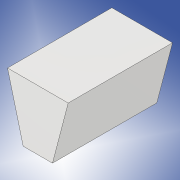
# Autodesk Inventor part: TA004
Saved by Autodesk Inventor 2017 (Build 210142000, 142)
## iProperties
Created: 2017-06-21
Part Number: TA004
Material: ABS Plastic
Document SubType Name: Modeling
Designer: zallen
Density: 1.06 g/cm^3
Appearance: CR White
Author: zallen
Autodesk Inventor part; units mm, degrees
ref_plane "YZ Plane" through (0, 0, 0) normal (1, 0, 0) x (0, 1, 0)
ref_plane "XZ Plane" through (0, 0, 0) normal (0, 1, 0) x (-1, 0, 0)
ref_plane "XY Plane" through (0, 0, 0) normal (0, 0, 1) x (1, 0, 0)
sketch "Sketch1" plane through (0, 0, 0) normal (0, 0, 1) x (1, 0, 0)
  line L0 (0, 0) -> (77.1779, 0)
  line L1 (0, 0) -> (-41.411, 158)
  line L2 (118.589, 158) -> (77.1779, 0)
  line L3 (38.589, 158) -> (38.589, 0) construction
  line L4 (-41.411, 158) -> (118.589, 158)
  dimension "d6" = 160
  dimension "d7" = 77.1779
  dimension "d8" = 158
  constraints: 10 end point, 2 horizontal, 2 midpoint, 1 vertical
  measures "d6" distance of L2.start L1.end
  measures "d7" distance of L0.start L0.end
  measures "d8" vertical distance of L0.end L2.start
extrude "Extrusion1" add sketch "Sketch1" along normal blind 275
body "Solid1"
